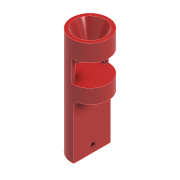
# Autodesk Inventor part: Tapered guide
Saved by Autodesk Inventor 2022 (Build 260153000, 153)
## iProperties
Created: 2022-02-16
Part Number: Tapered guide
Material: PC/ABS Plastic
Document SubType Name: Modeling
Designer: piers
Density: 0.357273 g/cm^3
Appearance: Red
Author: piers
Autodesk Inventor part; units mm, degrees
ref_plane "YZ Plane" through (0, 0, 0) normal (1, 0, 0) x (0, 1, 0)
ref_plane "XZ Plane" through (0, 0, 0) normal (0, 1, 0) x (-1, 0, 0)
ref_plane "XY Plane" through (0, 0, 0) normal (0, 0, 1) x (1, 0, 0)
sketch "Sketch1" plane through (0, 0, 0) normal (0, 1, 0) x (-1, 0, 0)
  circle A0 centre (0, 0) radius 13
  circle A1 centre (0, 0) radius 10.5
  line L0 (0, 13) -> (0, -13)
  point P0 (0, -10.5)
  point P1 (0, 10.5)
  dimension "d0" = 26
  dimension "d1" = 21
  constraints: 2 centre point, 2 coincident, 2 end point, 2 point on circle, 1 vertical
  measures "d0" diameter of A0
  measures "d1" diameter of A1
extrude "Extrusion1" add sketch "Sketch1" against normal blind 10
extrude "Extrusion2" add sketch "Sketch1" along normal blind 15.5 contours A0 L0 A1 picked at (12.058, 0.9643)
sketch "Sketch2" plane through (0, 15.5, 0) normal (0, 1, 0) x (1, 0, 0)
  circle A0 centre (0, 0) radius 13 projected
  circle A1 centre (0, 0) radius 10.5 projected
  circle A2 centre (0, 0) radius 5
  dimension "d6" = 10
  constraints: 1 centre point, 1 coincident
  measures "d6" diameter of A2
extrude "Extrusion3" add sketch "Sketch2" along normal blind 12 contours A0 | A1
extrude "Extrusion4" cut sketch "Sketch2" along normal blind 15 draft 25 contours A2
sketch "Sketch3" plane through (0, -10, 0) normal (0, -1, 0) x (1, 0, 0)
  line L0 (0, 0) -> (-1.5, 0)
  line L1 (-1.5, 0) -> (-1.5, -12.9132)
  circle A0 centre (0, 0) radius 13 projected
  line L2 (-1.5, 0) -> (-1.5, 12.9132)
  line L3 (0, 0) -> (0, -0.2769)
  line L4 (1.5, 0) -> (1.5, -12.9132)
  line L5 (1.5, 0) -> (1.5, 12.9132)
  point P0 (1.5, -12.9132)
  point P1 (1.5, 12.9132)
  dimension "d11" = 1.5
  constraints: 12 end point, 4 symmetric about line, 1 horizontal, 1 perpendicular, 1 vertical, 2 other
  measures "d11" distance of L0.start L0.end
extrude "Extrusion5" add sketch "Sketch3" along normal blind 38 contours L2 A0 L5 L4 L1
sketch "Sketch6" plane through (0, -10, 0) normal (0, -1, 0) x (1, 0, 0)
  line L0 (-1.5, -12.9132) -> (-1.5, 12.9132) projected
  arc A0 (-1.5, 12.9132) -> (-1.5, -12.9132) centre (0, 0) ccw projected
  arc A1 (1.5, -12.9132) -> (1.5, 12.9132) centre (0, 0) ccw projected
  line L1 (1.5, -12.9132) -> (1.5, 12.9132) projected
extrude "Extrusion7" add sketch "Sketch6" along normal blind 38 contours A0 L0
sketch "Sketch4" plane through (-1.5, -10, -12.9132) normal (-1, 0, 0) x (0, 0, 1)
  circle A0 centre (12.4097, -33) radius 1.5
  line L0 (25.8263, -38) -> (0, -38) projected
  circle A1 centre (12.4097, -6) radius 1.5
  point P0 (12.9132, 10)
  dimension "d14" = 5
  dimension "d17" = 3
  dimension "d18" = 3
  dimension "d19" = 27
  constraints: 2 centre point
  measures "d14" distance from line of A0.centre L0
  measures "d17" diameter of A0
  measures "d18" diameter of A1
  measures "d19" distance of A1.centre A0.centre
extrude "Extrusion6" cut sketch "Sketch4" along normal mid plane 30
chamfer "Chamfer1" distance 2 angle 45 1 edges at (1.5, -10, -6.4566)
sketch "Sketch7" plane through (0, -48, 0) normal (0, -1, 0) x (1, 0, 0)
  circle A0 centre (0, 0) radius 13 projected
  line L0 (-10.6184, 7.5) -> (-10.6184, -7.5)
  dimension "d25" = 15
  constraints: 2 end point, 2 point on circle, 1 vertical
  measures "d25" distance of L0.start L0.end
extrude "Extrusion8" cut sketch "Sketch7" against normal blind 38 contours L0 A0 picked at (-11.1206, 1.5629)
body "Solid1"
